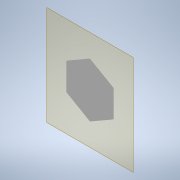
# Autodesk Inventor part: Mesh
Saved by Autodesk Inventor 2020.3 (Build 243373000, 373)
## iProperties
Created: 2020-07-07
Part Number: Mesh
Material: Generic
Document SubType Name: Modeling
Designer: Bruno
Density: 1 g/cm^3
Appearance: Default
Author: Bruno
Autodesk Inventor part; units mm, degrees
ref_plane "YZ Plane" through (0, 0, 0) normal (1, 0, 0) x (0, 1, 0)
ref_plane "XZ Plane" through (0, 0, 0) normal (0, 1, 0) x (-1, 0, 0)
ref_plane "XY Plane" through (0, 0, 0) normal (0, 0, 1) x (1, 0, 0)
ref_plane "Work Plane1" through (0, 0, 0) normal (0, 0, 1) x (1, 0, 0)
sketch "Sketch1" plane through (0, 0, 0) normal (0, 0, 1) x (1, 0, 0)
  line L0 (300, -173.2051) -> (0, -346.4102)
  line L1 (0, -346.4102) -> (-300, -173.2051)
  line L2 (-300, -173.2051) -> (-300, 173.2051)
  line L3 (-300, 173.2051) -> (0, 346.4102)
  line L4 (0, 346.4102) -> (300, 173.2051)
  line L5 (300, 173.2051) -> (300, -173.2051)
  point P0 (0, 0)
  point P1 (0, 0)
  dimension "d0" = 300
  constraints: 12 end point, 1 coincident, 1 vertical, 13 other
  measures "d0" distance from line of point (0, 0) L5
extrude "Extrusion1" add sketch "Sketch1" along normal blind 1
body "Solid1"
